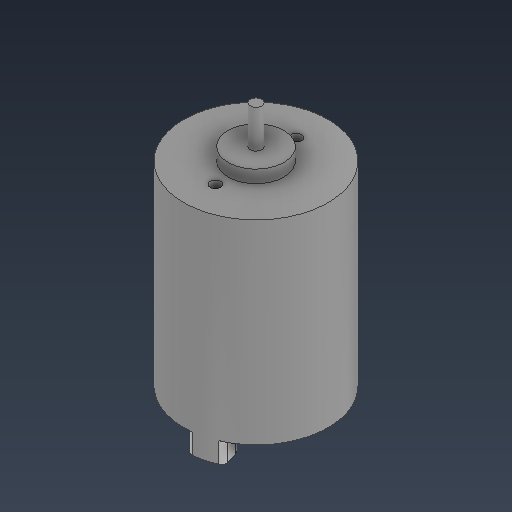
# Autodesk Inventor part: rs385
Saved by Autodesk Inventor 2027.1 (Build 311270010, 270A)
## iProperties
Created: 2025-03-30
Part Number: rs385
Material: Generic
Document SubType Name: Modeling
Designer: szymo
Density: 3.31598 g/cm^3
Appearance: Default
Mass: 80 g
Surface Area: 50.2469 cm^2
Volume: 24.1256 cm^3
Author: szymo
Autodesk Inventor part; units mm, degrees
ref_plane "YZ Plane" through (0, 0, 0) normal (1, 0, 0) x (0, 1, 0)
ref_plane "XZ Plane" through (0, 0, 0) normal (0, 1, 0) x (-1, 0, 0)
ref_plane "XY Plane" through (0, 0, 0) normal (0, 0, 1) x (1, 0, 0)
sketch "Sketch1" plane through (0, 0, 0) normal (0, 1, 0) x (-1, 0, 0)
  circle A0 centre (0, 0) radius 14.25
  dimension "d0" = 28.5
  constraints: 1 centre point, 1 coincident
  measures "d0" diameter of A0
extrude "Extrusion1" add sketch "Sketch1" along normal blind 38.5
sketch "Sketch2" plane through (0, 38.5, 0) normal (0, 1, 0) x (1, 0, 0)
  circle A0 centre (0, 0) radius 5.5
  circle A1 centre (0, 0) radius 1.15
  circle A2 centre (0, 0) radius 8
  line L0 (0, -8) -> (0, 8)
  dimension "d3" = 11
  dimension "d6" = 2.3
  dimension "d9" = 16
  constraints: 6 coincident, 3 centre point, 2 end point, 2 point on circle, 1 midpoint, 1 vertical
  measures "d3" diameter of A0
  measures "d6" diameter of A1
  measures "d9" diameter of A2
extrude "Extrusion2" add sketch "Sketch2" along normal blind 2.5 contours A0 L0 A1 | L0 A1 A0 | L0 A1 | A1 L0
extrude "Extrusion3" add sketch "Sketch2" along normal blind 10 contours L0 A1 | A1 L0
hole "Hole1" at (0, 38.5, 8) at (0, 38.5, -8) direction (0, -1, 0) diameter 2.1129 depth 7.8 thread size "M2.6x0.45" class "6H" standard "ISO Metric profile"
sketch "Sketch3" plane through (0, 0, 0) normal (0, -1, 0) x (1, 0, 0)
  circle A0 centre (0, 0) radius 5.5
  dimension "d17" = 11
  constraints: 1 centre point, 1 coincident
  measures "d17" diameter of A0
extrude "Extrusion4" add sketch "Sketch3" along normal blind 4
sketch "Sketch4" plane through (0, 0, 0) normal (0, -1, 0) x (1, 0, 0)
  line L0 (-12.0122, 7.6623) -> (12.8258, 7.6623) construction
  line L1 (12.8258, 7.6623) -> (12.8258, -7.5309) construction
  line L2 (12.8258, -7.5309) -> (-12.0122, -7.5309) construction
  line L3 (-12.0122, -7.5309) -> (-12.0122, 7.6623) construction
  point P0 (0, 0)
  constraints: 2 other
sketch "Sketch5" plane through (0, 0, 0) normal (0, -1, 0) x (1, 0, 0)
  circle A0 centre (0, 8) radius 1.0564 projected
  circle A1 centre (0, -8) radius 1.0564 projected
  circle A2 centre (0, 0) radius 5.5 projected
  circle A3 centre (0, 0) radius 14.25 projected
  circle A4 centre (0, 0) radius 1.15 projected
  circle A5 centre (0, 0) radius 12
  circle A6 centre (0, 0) radius 11.5
  line L0 (4.5304, 11.112) -> (4.3999, 10.625)
  line L1 (1.6326, 11.8884) -> (1.5021, 11.4015)
  line L2 (-1.5021, -11.4015) -> (-1.6326, -11.8884)
  line L3 (-4.3999, -10.625) -> (-4.5304, -11.112)
  line L4 (3.6882, 13.7644) -> (-3.6882, -13.7644)
  line L5 (0, 14.25) -> (0, -14.25) construction
  circle A7 centre (0, 0) radius 14.25 projected
  dimension "d29" = 15
  dimension "d30" = 1.5
  dimension "d31" = 1.5
  dimension "d32" = 1.5
  dimension "d33" = 1.5
  dimension "d59" = 24
  dimension "d60" = 23
  constraints: 12 end point, 12 point on circle, 3 parallel, 2 centre point, 2 coincident, 2 point on line, 1 midpoint, 1 vertical
  measures "d29" angle of L5 L4
  measures "d30" distance between parallel lines of L0 L4
  measures "d31" distance between parallel lines of L4 L1
  measures "d32" distance between parallel lines of L2 L4
  measures "d33" distance between parallel lines of L4 L3
  measures "d59" diameter of A5
  measures "d60" diameter of A6
extrude "Extrusion5" add sketch "Sketch5" along normal up to surface (4 mm away) contours L4 A5 L0 A6 | A6 L1 A5 L4 | L4 A5 L3 A6 | A6 L2 A5 L4
sketch "Sketch6" plane through (0, 0, 0) normal (0, -1, 0) x (1, 0, 0)
  line L0 (-4.5304, -11.112) -> (-4.3999, -10.625) projected
  arc A0 (-4.5304, -11.112) -> (-1.6326, -11.8884) centre (0, 0) ccw projected
  line L1 (-1.5021, -11.4015) -> (-1.6326, -11.8884) projected
  arc A1 (-4.3999, -10.625) -> (-1.5021, -11.4015) centre (0, 0) ccw projected
  line L2 (1.5021, 11.4015) -> (1.6326, 11.8884) projected
  arc A2 (4.3999, 10.625) -> (1.5021, 11.4015) centre (0, 0) ccw projected
  line L3 (4.5304, 11.112) -> (4.3999, 10.625) projected
  arc A3 (4.5304, 11.112) -> (1.6326, 11.8884) centre (0, 0) ccw projected
  line L4 (0.4288, -9.9908) -> (-0.5089, -13.4904)
  arc A4 (-6.3045, -11.9375) -> (-0.5089, -13.4904) centre (0, 0) ccw
  line L5 (-6.3045, -11.9375) -> (-5.3668, -8.4379)
  arc A5 (-5.3668, -8.4379) -> (0.4288, -9.9908) centre (0, 0) ccw
  line L6 (-0.4288, 9.9908) -> (0.5089, 13.4904)
  arc A6 (6.3045, 11.9375) -> (0.5089, 13.4904) centre (0, 0) ccw
  line L7 (6.3045, 11.9375) -> (5.3668, 8.4379)
  arc A7 (5.3668, 8.4379) -> (-0.4288, 9.9908) centre (0, 0) ccw
  circle A8 centre (0, 0) radius 13.5
  circle A9 centre (0, 0) radius 10
  circle A10 centre (0, 0) radius 14.25 projected
  line L8 (-0.5089, -13.4904) -> (-0.7077, -14.2324)
  line L9 (-6.3045, -11.9375) -> (-6.5033, -12.6795)
  line L10 (0.5089, 13.4904) -> (0.7077, 14.2324)
  line L11 (6.3045, 11.9375) -> (6.5033, 12.6795)
  dimension "d61" = 1.5
  dimension "d62" = 1.5
  dimension "d63" = 3.4996
  constraints: 16 end point, 12 point on circle, 6 centre point, 4 collinear, 2 coincident, 2 concentric, 6 other
  measures "d61" radial gap between concentric circles of A1 A5
  measures "d62" radial gap between concentric circles of A2 A7
  measures "d63" vertical distance of L4.start L4.end
extrude "Extrusion6" add sketch "Sketch6" along normal up to surface (4 mm away) contours L4 A4 L5 A5 | L8 A10 L9 A4 | L6 A6 L7 A7 | L10 A10 L11 A6
fillet "Fillet1" radius 1 8 edges at (-5.3668, -2, -8.4379) (0.4288, -2, -9.9908) (-0.7077, -2, -14.2324) (-6.5033, -2, -12.6795) (5.3668, -2, 8.4379) (6.5033, -2, 12.6795) (-0.4288, -2, 9.9908) (0.7077, -2, 14.2324)
equation "\"d31\" = d30"
equation "\"d32\" = d30"
equation "\"d62\" = d61"
body "Solid1"
